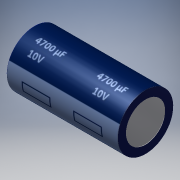
# Autodesk Inventor part: capacitor
Saved by Autodesk Inventor 2019 (Build 230136000, 136)
## iProperties
Created: 2020-03-05
Part Number: capacitor
Material: Generic
Document SubType Name: Modeling
Designer: ntb11189
Density: 1 g/cm^3
Appearance: Blue - Wall Paint - Glossy
Author: ntb11189
Autodesk Inventor part; units mm, degrees
ref_plane "YZ Plane" through (0, 0, 0) normal (1, 0, 0) x (0, 1, 0)
ref_plane "XZ Plane" through (0, 0, 0) normal (0, 1, 0) x (-1, 0, 0)
sketch "Sketch1" plane through (0, 0, 0) normal (1, 0, 0) x (0, 1, 0)
  circle A0 centre (0, 0) radius 6.35
  dimension "d0" = 6.35
  constraints: 1 centre point, 1 coincident
  measures "d0" radius of A0
extrude "Extrusion1" add sketch "Sketch1" along normal blind 25.5
ref_plane "Work Plane1" through (0, 0, 6.35) normal (0, 0, 1) x (1, 0, 0)
sketch "Sketch2" plane through (0, 0, 6.35) normal (0, 0, 1) x (1, 0, 0)
  line L0 (0.0077, -6.4259) -> (0.0077, 40.6963) construction
  line L1 (0.0077, 40.6963) -> (25.616, 40.6963) construction
  line L2 (25.616, 40.6963) -> (25.616, -6.4259) construction
  line L3 (25.616, -6.4259) -> (0.0077, -6.4259) construction
  point P0 (0, 0)
  constraints: 2 other
decal "Decal1"
sketch "Sketch3" plane through (25.5, 0, 0) normal (1, 0, 0) x (0, 0, -1)
  circle A0 centre (0, 0) radius 4.5
  dimension "d11" = 4.5
  constraints: 1 centre point, 1 coincident
  measures "d11" radius of A0
extrude "Extrusion2" cut sketch "Sketch3" against normal blind 0.1
body "Solid1"
